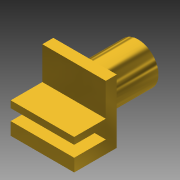
# Autodesk Inventor part: SMA_EdgeMale
Saved by Autodesk Inventor 2014 (Build 180170000, 170)
## iProperties
Created: 2015-01-07
Part Number: SMA_EdgeMale
Material: Generic
Document SubType Name: Modeling
Designer: Owner
Density: 1 g/cm^3
Appearance: Gold - Metal
Author: Owner
Autodesk Inventor part; units mm, degrees
ref_plane "YZ Plane" through (0, 0, 0) normal (1, 0, 0) x (0, 1, 0)
ref_plane "XZ Plane" through (0, 0, 0) normal (0, 1, 0) x (-1, 0, 0)
ref_plane "XY Plane" through (0, 0, 0) normal (0, 0, 1) x (1, 0, 0)
sketch "Sketch1" plane through (0, 0, 0) normal (0, 0, 1) x (1, 0, 0)
  line L0 (-4.8549, 2.8898) -> (4.6751, 2.8898)
  line L1 (4.6751, 2.8898) -> (4.6751, -6.6402)
  line L2 (4.6751, -6.6402) -> (-4.8549, -6.6402)
  line L3 (-4.8549, -6.6402) -> (-4.8549, 2.8898)
  point P0 (0, 0)
  dimension "d0" = 9.53
  dimension "d1" = 9.53
  constraints: 8 end point, 2 parallel, 1 horizontal, 1 perpendicular
  measures "d0" distance of L0.start L0.end
  measures "d1" distance of L0.end L1.end
extrude "Extrusion1" add sketch "Sketch1" along normal blind 1.65
sketch "Sketch2" plane through (4.6751, -6.6402, 0) normal (1, 0, 0) x (0, 0, -1)
  line L0 (-1.65, 0) -> (-1.65, 9.53) projected
  line L1 (-1.65, 3.59) -> (-6.4, 3.59)
  line L2 (-6.4, 3.59) -> (-6.4, 4.61)
  line L3 (-6.4, 4.61) -> (-1.65, 4.61)
  line L4 (-1.65, 4.61) -> (-1.65, 3.59)
  line L5 (-1.65, 0) -> (-6.4, 0)
  line L6 (-6.4, 0) -> (-6.4, 1.91)
  line L7 (-6.4, 1.91) -> (-1.65, 1.91)
  line L8 (-1.65, 1.91) -> (-1.65, 0)
  point P0 (0, 6.6402)
  dimension "d4" = 1.68
  dimension "d5" = 1.91
  dimension "d6" = 1.02
  dimension "d7" = 4.75
  dimension "d8" = 4.75
  constraints: 16 end point, 4 parallel, 2 horizontal, 2 perpendicular, 1 point on line
  measures "d4" distance between parallel lines of L1 L7
  measures "d5" distance between parallel lines of L5 L7
  measures "d6" distance between parallel lines of L3 L1
  measures "d7" distance between parallel lines of L0 L2
  measures "d8" distance between parallel lines of L0 L6
extrude "Extrusion2" add sketch "Sketch2" against normal blind 9.53
sketch "Sketch3" plane through (0, 0, 0) normal (0, 0, -1) x (-1, 0, 0)
  circle A0 centre (0, -1.8752) radius 3.05
  point P0 (0, 0)
  dimension "d11" = 6.1
  constraints: 1 centre point
  measures "d11" diameter of A0
extrude "Extrusion3" add sketch "Sketch3" along normal blind 7.88
body "Solid1"
